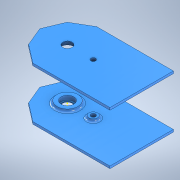
# Autodesk Inventor part: obudowa przekładni
Saved by Autodesk Inventor 2021 (Build 250183000, 183)
## iProperties
Created: 2021-06-25
Part Number: obudowa przekładni
Material: Generic
Document SubType Name: Modeling
Designer: Łukasz
Density: 1 g/cm^3
Appearance: Cyan
Author: Łukasz
Autodesk Inventor part; units mm, degrees
ref_plane "YZ Plane" through (0, 0, 0) normal (1, 0, 0) x (0, 1, 0)
ref_plane "XZ Plane" through (0, 0, 0) normal (0, 1, 0) x (-1, 0, 0)
ref_plane "XY Plane" through (0, 0, 0) normal (0, 0, 1) x (1, 0, 0)
sketch "Sketch1" plane through (0, 0, 0) normal (0, 1, 0) x (-1, 0, 0)
  circle A0 centre (0, 0) radius 11
  line L0 (0, -45) -> (-3.931, -45)
  line L1 (-3.2842, 50) -> (0, 50)
  line L2 (37.8352, 0) -> (26.6415, 27.0241)
  line L3 (26.6415, 27.0241) -> (-0.6792, 48)
  line L4 (-0.6792, 48) -> (-130, 48)
  line L5 (-130, -43) -> (-0.5468, -43)
  line L6 (-0.5468, -43) -> (26.692, -26.9021)
  line L7 (26.692, -26.9021) -> (37.8352, 0)
  line L8 (-130, 48) -> (-130, -43)
  line L9 (28.2843, -28.2843) -> (25.4178, -29.9783)
  line L10 (3.3842, -43) -> (0, -45)
  line L11 (40, 0) -> (38.9176, -2.6131)
  line L12 (29.5585, -25.2081) -> (28.2843, -28.2843)
  line L13 (28.2843, 28.2843) -> (29.8157, 24.587)
  line L14 (38.9176, 2.6131) -> (40, 0)
  line L15 (0, 50) -> (2.605, 48)
  line L16 (25.11, 30.7214) -> (28.2843, 28.2843)
  circle A1 centre (-44.3, 0) radius 4
  line L17 (1.9138, -52) -> (-130, -52)
  line L18 (-130, 57) -> (2.3773, 57)
  line L19 (2.3773, 57) -> (34.034, 32.695)
  line L20 (34.034, 32.695) -> (47.5767, 0)
  line L21 (47.5767, 0) -> (33.8573, -33.1217)
  line L22 (33.8573, -33.1217) -> (1.9138, -52)
  line L23 (-130, -52) -> (-130, -43)
  line L24 (-130, 48) -> (-130, 57)
  line L25 (-139, -45) -> (-139, -43)
  line L26 (-139, 48) -> (-139, 50)
  dimension "d7" = 8
  dimension "d8" = 44.3
  dimension "d13" = 22
  dimension "d14" = 9
  constraints: 54 end point, 15 point on line, 2 centre point, 2 perpendicular, 3 other
  measures "d7" diameter of A1
  measures "d8" distance of point (0, 0) A1.centre
  measures "d13" diameter of A0
  measures "d14" distance between parallel lines of L5 L17
extrude "Extrusion1" add sketch "Sketch1" along normal blind 4
sketch "Sketch2" plane through (0, 4, 0) normal (0, 1, 0) x (1, 0, 0)
  circle A0 centre (0, 0) radius 11 projected
  circle A1 centre (0, 0) radius 18
  circle A2 centre (44.3, 0) radius 4 projected
  circle A3 centre (44.3, 0) radius 7.5
  dimension "d3" = 36
  dimension "d9" = 15
  constraints: 2 centre point, 2 coincident
  measures "d3" diameter of A1
  measures "d9" diameter of A3
extrude "Extrusion2" add sketch "Sketch2" along normal blind 4
sketch "Sketch3" plane through (0, 4, 0) normal (0, 1, 0) x (1, 0, 0)
  point P0 (0, 0)
fillet "Fillet3" radius 4 2 edges at (36.8, 4, 0) (-18, 4, 0)
ref_plane "Work Plane1" through (0, 45.5, 0) normal (0, -1, 0) x (1, 0, 0)
mirror "Mirror1" about plane through (0, 45.5, 0) normal (0, -1, 0) of "Extrusion1", "Extrusion2", "Fillet3"
sketch "Sketch4" plane through (0, 0, 0) normal (0, -1, 0) x (1, 0, 0)
  point P0 (0, 0)
sketch "Sketch5" plane through (0, 0, 0) normal (0, -1, 0) x (1, 0, 0)
  circle A0 centre (0, 0) radius 8
  circle A1 centre (0, 0) radius 11 projected
  dimension "d15" = 16
  constraints: 1 centre point, 1 coincident
  measures "d15" diameter of A0
extrude "Extrusion3" add sketch "Sketch5" against normal blind 1
sketch "Sketch6" plane through (-2.3773, 91, 57) normal (0, 1, 0) x (1, 0, 0)
  circle A0 centre (2.3773, 57) radius 11 projected
  circle A1 centre (2.3773, 57) radius 8 projected
extrude "Extrusion4" add sketch "Sketch6" against normal blind 1
body "Solid1"
